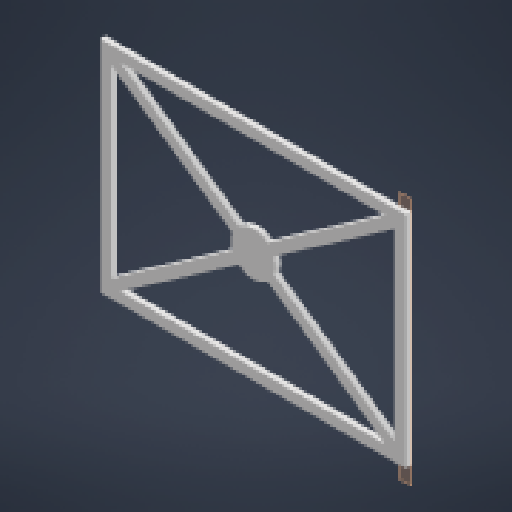
# Autodesk Inventor part: bracing
Saved by Autodesk Inventor 2026.3 (Build 303398000, 398)
## iProperties
Created: 2026-05-06
Part Number: bracing
Material: Generic
Document SubType Name: Modeling
Designer: frede
Density: 1 g/cm^3
Appearance: Default
Author: frede
Autodesk Inventor part; units mm, degrees
ref_plane "YZ Plane" through (0, 0, 0) normal (1, 0, 0) x (0, 1, 0)
ref_plane "XZ Plane" through (0, 0, 0) normal (0, 1, 0) x (-1, 0, 0)
ref_plane "XY Plane" through (0, 0, 0) normal (0, 0, 1) x (1, 0, 0)
ref_plane "Work Plane1" through (0, 0, 0) normal (0, 0, 1) x (1, 0, 0)
sketch "Sketch1" plane through (0, 0, 0) normal (0, 0, 1) x (1, 0, 0)
  line L0 (5, -5) -> (5, -95)
  line L1 (-134, -5) -> (-134, -95)
  line L2 (5, -95) -> (-134, -95)
  line L3 (-134, -5) -> (5, -5)
  line L4 (5, 0) -> (5, -102.9406) projected
  line L5 (0, -10) -> (-129, -10)
  line L6 (-129, -10) -> (-129, -90)
  line L7 (-129, -90) -> (0, -90)
  line L8 (0, -90) -> (0, -10)
  line L9 (0, -10) -> (-129, -90)
  line L10 (0, -90) -> (-129, -10)
  circle A0 centre (-64.5, -50) radius 10
  circle A1 centre (-64.5, -50) radius 2.5
  line L11 (0, -87.0583) -> (-124.2565, -10)
  line L12 (-4.7435, -90) -> (-129, -12.9417)
  line L13 (-124.2565, -90) -> (0, -12.9417)
  line L14 (-129, -87.0583) -> (-4.7435, -10)
  point P0 (0, 0)
  point P1 (-44.6355, -59.3773)
  point P2 (-42.6839, -66.4711)
  point P3 (-54.9538, -47.0216)
  point P4 (0, -17.9417)
  point P5 (-54.9538, -52.9784)
  point P6 (-74.0462, -47.0216)
  point P7 (-71.411, -42.7724)
  point P8 (-71.411, -57.2276)
  point P9 (-57.589, -57.2276)
  point P10 (-59.7565, -50)
  point P11 (-74.0462, -52.9784)
  point P12 (-57.589, -42.7724)
  dimension "d0" = 90
  dimension "d1" = 139
  dimension "d2" = 0
  dimension "d3" = 80
  dimension "d4" = 129
  dimension "d5" = 5
  dimension "d6" = 5
  dimension "d7" = 20
  dimension "d8" = 5
  dimension "d14" = 5
  constraints: 28 end point, 10 point on line, 8 parallel, 4 tangent, 2 centre point, 2 horizontal, 1 coincident, 1 midpoint, 1 perpendicular
  measures "d0" distance between parallel lines of L3 L2
  measures "d1" distance between parallel lines of L1 L0
  measures "d2" distance between parallel lines of L4 L0
  measures "d3" distance of L6.end L5.end
  measures "d4" distance between parallel lines of L6 L8
  measures "d5" distance between parallel lines of L2 L7
  measures "d6" distance between parallel lines of L0 L8
  measures "d7" diameter of A0
  measures "d8" diameter of A1
  measures "d14" distance from line of point (0, 0) L3
extrude "Extrusion1" add sketch "Sketch1" along normal blind 2.5 contours L0 L2 L1 L3 | L9 A0 L14 L5 | L8 L13 A0 L9 | A0 L13 L11 L9 | L9 L11 L14 A0 | L11 A0 L10 L5 | L14 L11 A0 | L8 L10 A0 L11 | A0 L11 L13 | L11 L13 L10 A1 L9 | L9 A1 L11 | L10 A0 L12 L6 | L11 L14 L10 A0 | L11 A1 L14 | L7 L12 A0 L10 | A0 L10 L13 L11 | A1 L10 L9 | L9 L10 A1 | L10 L14 L12 A0 | A1 L10 L14 | A0 L12 L13 L10 | L13 A1 L10 | L10 A1 L9 | L9 A1 L10 | L14 A0 L9 L6 | L12 L14 A0 | L10 A1 L9 L12 L14 | L7 L9 A0 L13 | A0 L13 L12 | L13 L12 A1 | A1 L12 L9 | L14 L12 L9 A0 | A0 L9 L12 L13
fillet "Fillet1" radius 5 20 edges at (-4.7435, -90, 1.25) (0, -87.0583, 1.25) (-124.2565, -90, 1.25) (-129, -87.0583, 1.25) (-129, -12.9417, 1.25) (-124.2565, -10, 1.25) (-4.7435, -10, 1.25) (0, -12.9417, 1.25) (-54.9538, -52.9784, 1.25) (-57.589, -57.2276, 1.25) (-71.411, -57.2276, 1.25) (-74.0462, -52.9784, 1.25) (-74.0462, -47.0216, 1.25) (-71.411, -42.7724, 1.25) (-57.589, -42.7724, 1.25) (5, -95, 1.25) (-134, -95, 1.25) (-134, -5, 1.25) (5, -5, 1.25) (-54.9538, -47.0216, 1.25)
equation "\"d5\" = -0.5 * d3 + 0.5 * d0"
equation "\"d6\" = -0.5 * d4 + 0.5 * d1"
body "Solid1"
